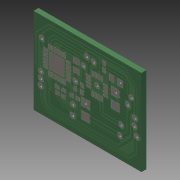
# Autodesk Inventor part: Sensor_module_uCMotionBoard_PCB
Saved by Autodesk Inventor 2013 (Build 170138000, 138)
## iProperties
Created: 2015-07-01
Part Number: Sensor_module_uCMotionBoard_PCB
Material: Ogólny
Document SubType Name: Modeling
Designer: terg
Density: 1 g/cm^3
Author: terg
Autodesk Inventor part; units mm, degrees
ref_plane "YZ Plane" through (0, 0, 0) normal (1, 0, 0) x (0, 1, 0)
ref_plane "XZ Plane" through (0, 0, 0) normal (0, 1, 0) x (-1, 0, 0)
ref_plane "XY Plane" through (0, 0, 0) normal (0, 0, 1) x (1, 0, 0)
sketch "Szkic1" plane through (0, 0, 0) normal (0, 1, 0) x (-1, 0, 0)
  line L0 (0, 0) -> (17.594, 0)
  line L1 (17.594, 0) -> (17.594, 14)
  line L2 (17.594, 14) -> (0, 14)
  line L3 (0, 14) -> (0, 0)
  dimension "d0" = 17.594
  dimension "d1" = 14
  constraints: 8 end point, 2 parallel, 1 horizontal, 1 perpendicular
  measures "d0" distance of L2.end L1.end
  measures "d1" distance of L1.end L0.end
extrude "Wyciągnięcie proste1" add sketch "Szkic1" along normal blind 0.8
sketch "Szkic2" plane through (0, 0.8, 0) normal (0, 1, 0) x (1, 0, 0)
  line L0 (0, 0) -> (-17.594, 0) projected
  line L1 (-17.594, 0) -> (-17.594, -14) projected
  line L2 (-17.594, -14) -> (0, -14) projected
  line L3 (0, -14) -> (0, 0) projected
  line L4 (-17.5939, 0) -> (-0.0001, 0) construction
  line L5 (-0.0001, 0) -> (-0.0001, -14) construction
  line L6 (-0.0001, -14) -> (-17.5939, -14) construction
  line L7 (-17.5939, -14) -> (-17.5939, 0) construction
  dimension "d158" = 0.0001
  dimension "d159" = 0
  dimension "d160" = 0
  dimension "d161" = 0.0001
  constraints: 2 other
  measures "d158" distance between parallel lines of L3 L5
  measures "d159" distance between parallel lines of L0 L4
  measures "d160" distance between parallel lines of L2 L6
  measures "d161" distance between parallel lines of L1 L7
decal "Pokrycie bitmapą1"
sketch "Szkic3" plane through (0, 0, 0) normal (0, -1, 0) x (1, 0, 0)
  line L0 (0, 0) -> (-17.594, 0) projected
  line L1 (0, 14) -> (0, 0) projected
  line L2 (-17.594, 14) -> (0, 14) projected
  line L3 (-17.594, 0) -> (-17.594, 14) projected
  line L4 (0.0133, 0) -> (-17.6073, 0) construction
  line L5 (-17.6073, 0) -> (-17.6073, 14) construction
  line L6 (-17.6073, 14) -> (0.0133, 14) construction
  line L7 (0.0133, 14) -> (0.0133, 0) construction
  dimension "d129" = -0.0133
  dimension "d130" = 0
  dimension "d131" = 0
  dimension "d134" = -0.0133
  constraints: 2 other
  measures "d129" distance between parallel lines of L3 L5
  measures "d130" distance between parallel lines of L2 L6
  measures "d131" distance between parallel lines of L0 L4
  measures "d134" distance between parallel lines of L1 L7
decal "Pokrycie bitmapą2"
sketch "Szkic4" plane through (0, 0, 0) normal (0, -1, 0) x (1, 0, 0)
  point P0 (-16.2702, 10.7609)
  point P1 (-8.9159, 11.8659)
  point P2 (-7.7882, 11.6457)
  point P3 (-9.4505, 10.28)
  point P4 (-10.7547, 7.5098)
  point P5 (-7.217, 8.6058)
  point P6 (-3.4608, 10.9118)
  point P7 (-4.1733, 9.1666)
  point P8 (-1.6325, 9.6914)
  point P9 (-2.2361, 8.3912)
  point P10 (-1.0276, 7.0921)
  point P11 (-1.1503, 5.8912)
  point P12 (-0.7724, 4.5937)
  point P13 (-3.3128, 5)
  point P14 (-3.4982, 3.3912)
  point P15 (-9.0919, 5.1642)
  point P16 (-11.1721, 3.9666)
  point P17 (-11.1983, 2.3896)
  point P18 (-16.4055, 3.9472)
  point P19 (-16.3754, 5.0322)
  point P20 (-16.4027, 6.0596)
hole "Otwór1" at (-16.2702, 0, 10.7609) at (-8.9159, 0, 11.8659) at (-7.7882, 0, 11.6457) at (-9.4505, 0, 10.28) at (-10.7547, 0, 7.5098) at (-7.217, 0, 8.6058) at (-3.4608, 0, 10.9118) at (-4.1733, 0, 9.1666) at (-1.6325, 0, 9.6914) at (-2.2361, 0, 8.3912) at (-1.0276, 0, 7.0921) at (-1.1503, 0, 5.8912) at (-0.7724, 0, 4.5937) at (-3.3128, 0, 5) at (-3.4982, 0, 3.3912) at (-9.0919, 0, 5.1642) at (-11.1721, 0, 3.9666) at (-11.1983, 0, 2.3896) at (-16.4055, 0, 3.9472) at (-16.3754, 0, 5.0322) at (-16.4027, 0, 6.0596) direction (0, 1, 0) diameter 0.4 depth 8
equation "\"d158\" = d161"
equation "\"d129\" = d134"
